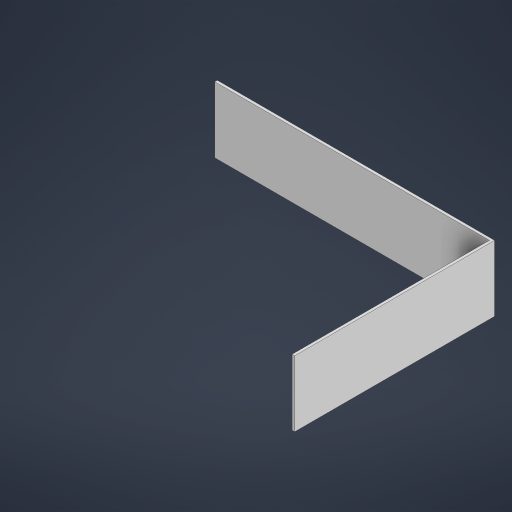
# Autodesk Inventor part: Piastrelle cucina
Saved by Autodesk Inventor 2024.2 (Build 282272000, 272)
## iProperties
Created: 2025-08-13
Part Number: Piastrelle cucina
Material: Generic
Document SubType Name: Modeling
Designer: Luca
Density: 1 g/cm^3
Appearance: Default
Author: Luca
Autodesk Inventor part; units mm, degrees
ref_plane "YZ Plane" through (0, 0, 0) normal (1, 0, 0) x (0, 1, 0)
ref_plane "XZ Plane" through (0, 0, 0) normal (0, 1, 0) x (-1, 0, 0)
ref_plane "XY Plane" through (0, 0, 0) normal (0, 0, 1) x (1, 0, 0)
sketch "Sketch1" plane through (0, 0, 0) normal (0, 1, 0) x (-1, 0, 0)
  line L0 (2150, 0) -> (0, 0)
  line L1 (0, 0) -> (0, 1550)
  line L2 (0, 1550) -> (20, 1550)
  line L3 (20, 1550) -> (20, 20)
  line L4 (20, 20) -> (2150, 20)
  line L5 (2150, 20) -> (2150, 0)
  dimension "d0" = 2150
  dimension "d1" = 1550
  dimension "d2" = 20
  constraints: 12 end point, 6 perpendicular, 1 coincident, 1 horizontal
  measures "d0" distance of L0.start L0.end
  measures "d1" distance of L0.end L1.end
  measures "d2" distance between parallel lines of L4 L0
extrude "Extrusion1" add sketch "Sketch1" along normal blind 510
body "Solid1"
